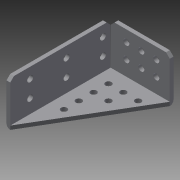
# Autodesk Inventor part: Chassis_BumperAttachment Bruh
Saved by Autodesk Inventor 2014 (Build 180170000, 170)
## iProperties
Created: 2016-01-25
Part Number: Chassis_BumperAttachment Bruh
Material: Generic
Document SubType Name: Modeling
Designer: owensm
Density: 1 g/cm^3
Appearance: Default
Author: owensm
Autodesk Inventor part; units mm, degrees
ref_plane "YZ Plane" through (0, 0, 0) normal (1, 0, 0) x (0, 1, 0)
ref_plane "XZ Plane" through (0, 0, 0) normal (0, 1, 0) x (-1, 0, 0)
ref_plane "XY Plane" through (0, 0, 0) normal (0, 0, 1) x (1, 0, 0)
sketch "Sketch1" plane through (0, 0, 0) normal (0, 1, 0) x (-1, 0, 0)
  line L0 (2.0728, 0) -> (87.1628, 0)
  line L1 (87.1628, 0) -> (87.1628, -50.165)
  line L2 (87.1628, -50.165) -> (2.0728, -50.165)
  line L3 (2.0728, -50.165) -> (2.0728, 0)
  line L4 (87.1628, -50.165) -> (2.0728, 0)
  point P0 (0, 0)
  dimension "d0" = 85.09
  dimension "d1" = 50.165
  constraints: 10 end point, 2 parallel, 1 horizontal, 1 perpendicular
  measures "d0" distance of L1.end L2.end
  measures "d1" distance of L0.end L1.end
extrude "Extrusion1" add sketch "Sketch1" along normal blind 3.175 contours L0 L1 L4
sketch "Sketch2" plane through (0, 3.175, 0) normal (0, 1, 0) x (1, 0, 0)
  line L0 (-87.1628, 0) -> (-2.0728, 0) projected
  line L1 (-87.1628, 0) -> (-90.3378, 0)
  line L2 (-90.3378, 0) -> (-90.3378, 50.165)
  line L3 (-90.3378, 50.165) -> (-87.1628, 50.165)
  line L4 (-87.1628, 50.165) -> (-87.1628, 0)
  line L5 (-87.1628, 0) -> (-2.0728, 0)
  line L6 (-2.0728, 0) -> (-2.0728, -3.175)
  line L7 (-2.0728, -3.175) -> (-87.1628, -3.175)
  line L8 (-87.1628, -3.175) -> (-87.1628, 0)
  line L9 (-90.3378, 0) -> (-87.1628, 0)
  line L10 (-87.1628, 0) -> (-87.1628, -3.175)
  line L11 (-87.1628, -3.175) -> (-90.3378, -3.175)
  line L12 (-90.3378, -3.175) -> (-90.3378, 0)
  point P0 (0, 0)
  dimension "d4" = 3.175
  dimension "d5" = 3.175
  constraints: 24 end point, 6 parallel, 3 horizontal, 3 perpendicular
  measures "d4" distance between parallel lines of L4 L2
  measures "d5" distance between parallel lines of L0 L7
extrude "Extrusion2" add sketch "Sketch2" along normal blind 34.7726 contours L1 L2 L3 L4 | L0 L6 L7 L8
sketch "Sketch3" plane through (0, 37.9476, 0) normal (0, 1, 0) x (1, 0, 0)
  line L0 (-87.1628, 0) -> (-90.3378, 0)
  line L1 (-90.3378, 0) -> (-90.3378, -3.175)
  line L2 (-90.3378, -3.175) -> (-87.1628, -3.175)
  line L3 (-87.1628, -3.175) -> (-87.1628, 0)
  point P0 (0, 0)
  dimension "d8" = 3.175
  constraints: 8 end point, 2 parallel, 1 horizontal, 1 perpendicular
  measures "d8" distance of L2.end L1.end
extrude "Extrusion3" add sketch "Sketch3" against normal blind 34.7726
sketch "Sketch4" plane through (0, 3.175, 0) normal (0, -1, 0) x (1, 0, 0)
  line L0 (-87.1628, 0) -> (-2.0728, 0) projected
  line L1 (-2.0728, 3.175) -> (-2.0728, 0) projected
  line L2 (-2.0728, 3.175) -> (-90.3378, 3.175) projected
  line L3 (-90.3378, -50.165) -> (-90.3378, 3.175) projected
  line L4 (-87.1628, -50.165) -> (-90.3378, -50.165) projected
  line L5 (-87.1628, -50.165) -> (-87.1628, 0) projected
  point P0 (0, 0)
extrude "Extrusion4" add sketch "Sketch4" along normal blind 3.175
fillet "Fillet1" radius 3.175 2 edges at (-46.2053, 0, 3.175) (-90.3378, 0, -23.495)
sketch "Sketch5" plane through (0, 0, 0) normal (0, -1, 0) x (1, 0, 0)
  line L0 (-87.0358, -0.127) -> (-90.3378, -0.127)
  line L1 (-90.3378, -0.127) -> (-90.3378, 3.175)
  line L2 (-90.3378, 3.175) -> (-87.0358, 3.175)
  line L3 (-87.0358, 3.175) -> (-87.0358, -0.127)
  line L4 (-90.3378, 0) -> (-90.3378, -50.165) projected
  line L5 (-2.0728, 3.175) -> (-87.1628, 3.175) projected
  point P0 (0, 0)
  dimension "d22" = 3.302
  dimension "d23" = 3.302
  dimension "d24" = 0
  dimension "d25" = 0
  constraints: 8 end point, 2 parallel, 1 horizontal, 1 perpendicular
  measures "d22" distance of L1.end L2.end
  measures "d23" distance of L2.end L0.start
  measures "d24" distance between parallel lines of L4 L1
  measures "d25" distance between parallel lines of L5 L2
extrude "Extrusion5" cut sketch "Sketch5" against normal blind 127
chamfer "Chamfer4" distance 3.175 angle 45 4 edges at (-2.0728, 37.9476, 1.5875) (-88.7503, 37.9476, -50.165) (-88.7503, 37.9476, -0.127) (-87.0358, 37.9476, 1.5875)
sketch "Sketch6" plane through (-87.1628, 3.175, -0.127) normal (1, 0, 0) x (0, 0, -1)
  line L0 (50.038, 0) -> (50.038, 31.5976) projected
  line L1 (3.175, 34.7726) -> (46.863, 34.7726) projected
  circle A0 centre (38.608, 25.3746) radius 2.54
  circle A1 centre (38.608, 12.6746) radius 2.54
  circle A2 centre (25.908, 25.3746) radius 2.54
  circle A3 centre (25.908, 12.6746) radius 2.54
  circle A4 centre (13.208, 25.3746) radius 2.54
  circle A5 centre (13.208, 12.6746) radius 2.54
  point P0 (-0.127, -3.175)
  dimension "d43" = 25.4
  dimension "d32" = 5.08
  dimension "d34" = 11.43
  dimension "d35" = 9.398
  dimension "d36" = 5.08
  dimension "d37" = 12.7
  dimension "d40" = 12.7
  constraints: 6 centre point, 1 horizontal, 8 other
  measures "d32" diameter of A0
  measures "d34" distance from line of L0 A0.centre
  measures "d35" distance from line of L1 A0.centre
  measures "d36" diameter of A1
  measures "d37" distance of A0.centre A1.centre
  measures "d40" distance of A0.centre A2.centre
extrude "Extrusion6" cut sketch "Sketch6" against normal blind 127
sketch "Sketch7" plane through (-2.0728, 3.175, 0) normal (0, 0, -1) x (-1, 0, 0)
  line L0 (3.175, 34.7726) -> (81.788, 34.7726) projected
  line L1 (84.963, 0) -> (0, 0) projected
  line L2 (84.963, 0) -> (84.963, 31.5976) projected
  circle A0 centre (78.613, 25.8826) radius 2.54
  circle A1 centre (47.752, 25.8826) radius 2.54
  circle A2 centre (16.891, 25.8826) radius 2.54
  circle A3 centre (78.613, 11.6586) radius 2.54
  circle A4 centre (47.752, 11.6586) radius 2.54
  circle A5 centre (16.891, 11.6586) radius 2.54
  point P0 (-2.0728, -3.175)
  dimension "d48" = 5.08
  dimension "d49" = 6.35
  dimension "d50" = 8.89
  dimension "d53" = 30.861
  dimension "d56" = 14.224
  constraints: 6 centre point, 1 horizontal, 1 vertical, 10 other
  measures "d48" diameter of A0
  measures "d49" distance from line of L2 A0.centre
  measures "d50" distance from line of A0.centre L0
  measures "d53" distance of A0.centre A1.centre
  measures "d56" distance of A0.centre A3.centre
extrude "Extrusion7" cut sketch "Sketch7" against normal blind 127
sketch "Sketch8" plane through (0, 3.175, 0) normal (0, 1, 0) x (1, 0, 0)
  line L0 (-87.0358, 0) -> (-2.0728, 0) projected
  line L1 (-87.1628, 50.165) -> (-87.1628, 0.127) projected
  circle A0 centre (-74.412, 36.0934) radius 2.54
  line L2 (-87.1628, 50.165) -> (-90.3378, 50.165) projected
  circle A1 centre (-61.839, 36.0934) radius 2.54
  circle A2 centre (-49.266, 36.0934) radius 2.54
  circle A3 centre (-36.693, 36.0934) radius 2.54
  circle A4 centre (-74.412, 23.5204) radius 2.54
  circle A5 centre (-61.839, 23.5204) radius 2.54
  circle A6 centre (-49.266, 23.5204) radius 2.54
  circle A7 centre (-36.693, 23.5204) radius 2.54
  circle A8 centre (-74.412, 10.9474) radius 2.54
  circle A9 centre (-61.839, 10.9474) radius 2.54
  circle A10 centre (-49.266, 10.9474) radius 2.54
  circle A11 centre (-36.693, 10.9474) radius 2.54
  point P0 (0, 0)
  dimension "d61" = 5.08
  dimension "d63" = 12.7508
  dimension "d64" = 14.0716
  dimension "d67" = 12.573
  dimension "d70" = 12.573
  constraints: 12 centre point, 1 horizontal, 1 vertical, 22 other
  measures "d61" diameter of A0
  measures "d63" distance from line of L1 A0.centre
  measures "d64" distance from line of L2 A0.centre
  measures "d67" distance of A0.centre A1.centre
  measures "d70" distance of A0.centre A4.centre
extrude "Extrusion8" cut sketch "Sketch8" against normal blind 127 contours A0 | A4 | A5 | A8 | A9 | A10 | A11
body "Solid1"
